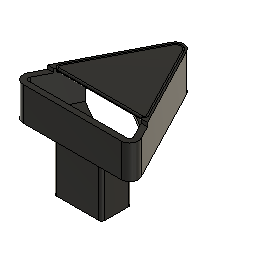
EMGmount (Autodesk Fusion 360 design; units mm, degrees)
Autodesk Fusion 360 part; units mm, degrees
sketch "Sketch5" plane through (0, 0, -6.0198) normal (0, 0, 1) x (-1, 0, 0)
  line L0 (-4.0409, -57.15) -> (2.9359, -57.15)
  line L1 (2.9359, -57.15) -> (3.9347, -56.1512)
  line L2 (3.9347, -56.1512) -> (3.9347, 6.35)
  line L3 (3.9347, 6.35) -> (-16.6393, 6.35)
  line L4 (-16.6393, 6.35) -> (-16.6393, -56.1512)
  line L5 (-16.6393, -56.1512) -> (-15.6405, -57.15)
  line L6 (-15.6405, -57.15) -> (-8.6637, -57.15)
  line L7 (-8.6637, -57.15) -> (-8.6637, -55.3466)
  arc A0 (-8.1557, -54.8386) -> (-8.6637, -55.3466) centre (-8.1557, -55.3466) ccw
  line L8 (-8.1557, -54.8386) -> (-4.5489, -54.8386)
  arc A1 (-4.0409, -55.3466) -> (-4.5489, -54.8386) centre (-4.5489, -55.3466) ccw
  line L9 (-4.0409, -55.3466) -> (-4.0409, -57.15)
  arc A2 (-8.1557, -42.1386) -> (-8.6637, -42.6466) centre (-8.1557, -42.6466) ccw
  line L10 (-8.1557, -42.1386) -> (-4.5489, -42.1386)
  arc A3 (-4.0409, -42.6466) -> (-4.5489, -42.1386) centre (-4.5489, -42.6466) ccw
  line L11 (-4.0409, -42.6466) -> (-4.0409, -46.2534)
  arc A4 (-4.5489, -46.7614) -> (-4.0409, -46.2534) centre (-4.5489, -46.2534) ccw
  line L12 (-4.5489, -46.7614) -> (-8.1557, -46.7614)
  arc A5 (-8.6637, -46.2534) -> (-8.1557, -46.7614) centre (-8.1557, -46.2534) ccw
  line L13 (-8.6637, -46.2534) -> (-8.6637, -42.6466)
  arc A6 (-8.1557, -29.4386) -> (-8.6637, -29.9466) centre (-8.1557, -29.9466) ccw
  line L14 (-8.1557, -29.4386) -> (-4.5489, -29.4386)
  arc A7 (-4.0409, -29.9466) -> (-4.5489, -29.4386) centre (-4.5489, -29.9466) ccw
  line L15 (-4.0409, -29.9466) -> (-4.0409, -33.5534)
  arc A8 (-4.5489, -34.0614) -> (-4.0409, -33.5534) centre (-4.5489, -33.5534) ccw
  line L16 (-4.5489, -34.0614) -> (-8.1557, -34.0614)
  arc A9 (-8.6637, -33.5534) -> (-8.1557, -34.0614) centre (-8.1557, -33.5534) ccw
  line L17 (-8.6637, -33.5534) -> (-8.6637, -29.9466)
  arc A10 (1.8011, -53.1114) -> (2.3091, -52.6034) centre (1.8011, -52.6034) ccw
  line L18 (1.8011, -53.1114) -> (-1.8057, -53.1114)
  arc A11 (-2.3137, -52.6034) -> (-1.8057, -53.1114) centre (-1.8057, -52.6034) ccw
  line L19 (-2.3137, -52.6034) -> (-2.3137, -48.9966)
  arc A12 (-1.8057, -48.4886) -> (-2.3137, -48.9966) centre (-1.8057, -48.9966) ccw
  line L20 (-1.8057, -48.4886) -> (1.8011, -48.4886)
  arc A13 (2.3091, -48.9966) -> (1.8011, -48.4886) centre (1.8011, -48.9966) ccw
  line L21 (2.3091, -48.9966) -> (2.3091, -52.6034)
  arc A14 (1.8011, -40.4114) -> (2.3091, -39.9034) centre (1.8011, -39.9034) ccw
  line L22 (1.8011, -40.4114) -> (-1.8057, -40.4114)
  arc A15 (-2.3137, -39.9034) -> (-1.8057, -40.4114) centre (-1.8057, -39.9034) ccw
  line L23 (-2.3137, -39.9034) -> (-2.3137, -36.2966)
  arc A16 (-1.8057, -35.7886) -> (-2.3137, -36.2966) centre (-1.8057, -36.2966) ccw
  line L24 (-1.8057, -35.7886) -> (1.8011, -35.7886)
  arc A17 (2.3091, -36.2966) -> (1.8011, -35.7886) centre (1.8011, -36.2966) ccw
  line L25 (2.3091, -36.2966) -> (2.3091, -39.9034)
  arc A18 (1.8011, -27.7114) -> (2.3091, -27.2034) centre (1.8011, -27.2034) ccw
  line L26 (1.8011, -27.7114) -> (-1.8057, -27.7114)
  arc A19 (-2.3137, -27.2034) -> (-1.8057, -27.7114) centre (-1.8057, -27.2034) ccw
  line L27 (-2.3137, -27.2034) -> (-2.3137, -23.5966)
  arc A20 (-1.8057, -23.0886) -> (-2.3137, -23.5966) centre (-1.8057, -23.5966) ccw
  line L28 (-1.8057, -23.0886) -> (1.8011, -23.0886)
  arc A21 (2.3091, -23.5966) -> (1.8011, -23.0886) centre (1.8011, -23.5966) ccw
  line L29 (2.3091, -23.5966) -> (2.3091, -27.2034)
  arc A22 (1.8011, -15.0114) -> (2.3091, -14.5034) centre (1.8011, -14.5034) ccw
  line L30 (1.8011, -15.0114) -> (-1.8057, -15.0114)
  arc A23 (-2.3137, -14.5034) -> (-1.8057, -15.0114) centre (-1.8057, -14.5034) ccw
  line L31 (-2.3137, -14.5034) -> (-2.3137, -10.8966)
  arc A24 (-1.8057, -10.3886) -> (-2.3137, -10.8966) centre (-1.8057, -10.8966) ccw
  line L32 (-1.8057, -10.3886) -> (1.8011, -10.3886)
  arc A25 (2.3091, -10.8966) -> (1.8011, -10.3886) centre (1.8011, -10.8966) ccw
  line L33 (2.3091, -10.8966) -> (2.3091, -14.5034)
  arc A26 (1.8011, -2.3114) -> (2.3091, -1.8034) centre (1.8011, -1.8034) ccw
  line L34 (1.8011, -2.3114) -> (-1.8057, -2.3114)
  arc A27 (-2.3137, -1.8034) -> (-1.8057, -2.3114) centre (-1.8057, -1.8034) ccw
  line L35 (-2.3137, -1.8034) -> (-2.3137, 1.8034)
  arc A28 (-1.8057, 2.3114) -> (-2.3137, 1.8034) centre (-1.8057, 1.8034) ccw
  line L36 (-1.8057, 2.3114) -> (1.8011, 2.3114)
  arc A29 (2.3091, 1.8034) -> (1.8011, 2.3114) centre (1.8011, 1.8034) ccw
  line L37 (2.3091, 1.8034) -> (2.3091, -1.8034)
  arc A30 (-10.8989, -53.1114) -> (-10.3909, -52.6034) centre (-10.8989, -52.6034) ccw
  line L38 (-10.8989, -53.1114) -> (-14.5057, -53.1114)
  arc A31 (-15.0137, -52.6034) -> (-14.5057, -53.1114) centre (-14.5057, -52.6034) ccw
  line L39 (-15.0137, -52.6034) -> (-15.0137, -48.9966)
  arc A32 (-14.5057, -48.4886) -> (-15.0137, -48.9966) centre (-14.5057, -48.9966) ccw
  line L40 (-14.5057, -48.4886) -> (-10.8989, -48.4886)
  arc A33 (-10.3909, -48.9966) -> (-10.8989, -48.4886) centre (-10.8989, -48.9966) ccw
  line L41 (-10.3909, -48.9966) -> (-10.3909, -52.6034)
  arc A34 (-10.8989, -40.4114) -> (-10.3909, -39.9034) centre (-10.8989, -39.9034) ccw
  line L42 (-10.8989, -40.4114) -> (-14.5057, -40.4114)
  arc A35 (-15.0137, -39.9034) -> (-14.5057, -40.4114) centre (-14.5057, -39.9034) ccw
  line L43 (-15.0137, -39.9034) -> (-15.0137, -36.2966)
  arc A36 (-14.5057, -35.7886) -> (-15.0137, -36.2966) centre (-14.5057, -36.2966) ccw
  line L44 (-14.5057, -35.7886) -> (-10.8989, -35.7886)
  arc A37 (-10.3909, -36.2966) -> (-10.8989, -35.7886) centre (-10.8989, -36.2966) ccw
  line L45 (-10.3909, -36.2966) -> (-10.3909, -39.9034)
  arc A38 (-10.8989, -27.7114) -> (-10.3909, -27.2034) centre (-10.8989, -27.2034) ccw
  line L46 (-10.8989, -27.7114) -> (-14.5057, -27.7114)
  arc A39 (-15.0137, -27.2034) -> (-14.5057, -27.7114) centre (-14.5057, -27.2034) ccw
  line L47 (-15.0137, -27.2034) -> (-15.0137, -23.5966)
  arc A40 (-14.5057, -23.0886) -> (-15.0137, -23.5966) centre (-14.5057, -23.5966) ccw
  line L48 (-14.5057, -23.0886) -> (-10.8989, -23.0886)
  arc A41 (-10.3909, -23.5966) -> (-10.8989, -23.0886) centre (-10.8989, -23.5966) ccw
  line L49 (-10.3909, -23.5966) -> (-10.3909, -27.2034)
  arc A42 (-10.8989, -15.0114) -> (-10.3909, -14.5034) centre (-10.8989, -14.5034) ccw
  line L50 (-10.8989, -15.0114) -> (-14.5057, -15.0114)
  arc A43 (-15.0137, -14.5034) -> (-14.5057, -15.0114) centre (-14.5057, -14.5034) ccw
  line L51 (-15.0137, -14.5034) -> (-15.0137, -10.8966)
  arc A44 (-14.5057, -10.3886) -> (-15.0137, -10.8966) centre (-14.5057, -10.8966) ccw
  line L52 (-14.5057, -10.3886) -> (-10.8989, -10.3886)
  arc A45 (-10.3909, -10.8966) -> (-10.8989, -10.3886) centre (-10.8989, -10.8966) ccw
  line L53 (-10.3909, -10.8966) -> (-10.3909, -14.5034)
  arc A46 (-10.8989, -2.3114) -> (-10.3909, -1.8034) centre (-10.8989, -1.8034) ccw
  line L54 (-10.8989, -2.3114) -> (-14.5057, -2.3114)
  arc A47 (-15.0137, -1.8034) -> (-14.5057, -2.3114) centre (-14.5057, -1.8034) ccw
  line L55 (-15.0137, -1.8034) -> (-15.0137, 1.8034)
  arc A48 (-14.5057, 2.3114) -> (-15.0137, 1.8034) centre (-14.5057, 1.8034) ccw
  line L56 (-14.5057, 2.3114) -> (-10.8989, 2.3114)
  arc A49 (-10.3909, 1.8034) -> (-10.8989, 2.3114) centre (-10.8989, 1.8034) ccw
  line L57 (-10.3909, 1.8034) -> (-10.3909, -1.8034)
  arc A50 (-8.6637, -8.1534) -> (-8.1557, -8.6614) centre (-8.1557, -8.1534) ccw
  line L58 (-8.6637, -8.1534) -> (-8.6637, -4.5466)
  arc A51 (-8.1557, -4.0386) -> (-8.6637, -4.5466) centre (-8.1557, -4.5466) ccw
  line L59 (-8.1557, -4.0386) -> (-4.5489, -4.0386)
  arc A52 (-4.0409, -4.5466) -> (-4.5489, -4.0386) centre (-4.5489, -4.5466) ccw
  line L60 (-4.0409, -4.5466) -> (-4.0409, -8.1534)
  arc A53 (-4.5489, -8.6614) -> (-4.0409, -8.1534) centre (-4.5489, -8.1534) ccw
  line L61 (-4.5489, -8.6614) -> (-8.1557, -8.6614)
  arc A54 (-8.1557, -16.7386) -> (-8.6637, -17.2466) centre (-8.1557, -17.2466) ccw
  line L62 (-8.1557, -16.7386) -> (-4.5489, -16.7386)
  arc A55 (-4.0409, -17.2466) -> (-4.5489, -16.7386) centre (-4.5489, -17.2466) ccw
  line L63 (-4.0409, -17.2466) -> (-4.0409, -20.8534)
  arc A56 (-4.5489, -21.3614) -> (-4.0409, -20.8534) centre (-4.5489, -20.8534) ccw
  line L64 (-4.5489, -21.3614) -> (-8.1557, -21.3614)
  arc A57 (-8.6637, -20.8534) -> (-8.1557, -21.3614) centre (-8.1557, -20.8534) ccw
  line L65 (-8.6637, -20.8534) -> (-8.6637, -17.2466)
  line L66 (3.9347, 5.08) -> (3.9347, -5.08)
  line L67 (2.6647, -6.35) -> (-15.3693, -6.35)
  line L68 (-16.6393, -5.08) -> (-16.6393, 5.08)
  line L69 (-15.3693, 6.35) -> (2.6647, 6.35)
  arc A58 (2.6647, -6.35) -> (3.9347, -5.08) centre (2.6647, -5.08) ccw
  arc A59 (3.9347, 5.08) -> (2.6647, 6.35) centre (2.6647, 5.08) ccw
  arc A60 (-16.6393, -5.08) -> (-15.3693, -6.35) centre (-15.3693, -5.08) ccw
  arc A61 (-15.3693, 6.35) -> (-16.6393, 5.08) centre (-15.3693, 5.08) ccw
  point P0 (3.9347, 6.35)
  point P1 (3.9347, -6.35)
  dimension "d56" = 12.7
  dimension "d57" = 1.27
  constraint coincident P0 L2.end
  constraint coincident L2 P1
  constraint perpendicular L4 L67
  constraint coincident P1 L66
  constraint coincident P1 L67
  constraint tangent L66 A58
  constraint tangent L67 A58
  constraint coincident P0 L66
  constraint coincident P0 L69
  constraint tangent L66 A59
  constraint tangent L69 A59
  constraint equal A58 A59
  constraint tangent L67 A60
  constraint tangent L68 A60
  constraint equal A58 A60
  constraint tangent L68 A61
  constraint tangent L69 A61
  constraint equal A58 A61
  measures "d56" distance of P0 P1
  measures "d57" radius of A58
extrude "Extrude8" add sketch "Sketch5" along normal blind 22.225 contours L2 L3 L4 L58 A51 L59 A52 L60 L66 L67 L68 L69 A58 A59 A60 A61 | L58 A51 L59 A52 L60 L67 | A26 L34 A27 L35 A28 L36 A29 L37 | A46 L54 A47 L55 A48 L56 A49 L57 makes body 1
sketch "Sketch9" plane through (0, 0, 16.2052) normal (0, 0, 1) x (-1, 0, 0)
  arc A0 (3.9347, 5.08) -> (2.6647, 6.35) centre (2.6647, 5.08) ccw
  line L0 (2.6647, 6.35) -> (-15.3693, 6.35)
  arc A1 (-15.3693, 6.35) -> (-16.6393, 5.08) centre (-15.3693, 5.08) ccw
  line L1 (-16.6393, 5.08) -> (-16.6393, -5.08)
  arc A2 (-16.6393, -5.08) -> (-15.3693, -6.35) centre (-15.3693, -5.08) ccw
  line L2 (-15.3693, -6.35) -> (2.6647, -6.35)
  arc A3 (2.6647, -6.35) -> (3.9347, -5.08) centre (2.6647, -5.08) ccw
  line L3 (3.9347, -5.08) -> (3.9347, 5.08)
  line L4 (-6.3523, 6.35) -> (-27.2641, 6.35)
  line L5 (-6.3523, 6.35) -> (14.5594, 6.35)
  line L6 (-6.3523, 6.35) -> (-6.3523, -83.9563)
  line L7 (15.6871, 4.4958) -> (-5.2247, -35.8693)
  line L8 (-7.48, -35.8693) -> (-28.3917, 4.4958)
  arc A4 (-7.48, -35.8693) -> (-5.2247, -35.8693) centre (-6.3523, -35.2851) ccw
  arc A5 (-27.2641, 6.35) -> (-28.3917, 4.4958) centre (-27.2641, 5.08) ccw
  arc A6 (15.6871, 4.4958) -> (14.5594, 6.35) centre (14.5594, 5.08) ccw
  line L9 (-6.3523, 8.7312) -> (-27.2641, 8.7312)
  arc A7 (-27.2641, 8.7312) -> (-30.5061, 3.4004) centre (-27.2641, 5.08) ccw
  line L10 (-9.5943, -36.9647) -> (-30.5061, 3.4004)
  arc A8 (-9.5943, -36.9647) -> (-3.1103, -36.9647) centre (-6.3523, -35.2851) ccw
  line L11 (17.8014, 3.4004) -> (-3.1103, -36.9647)
  arc A9 (17.8014, 3.4004) -> (14.5594, 8.7313) centre (14.5594, 5.08) ccw
  line L12 (-6.3523, 8.7312) -> (14.5594, 8.7312)
  point P0 (-29.3523, 6.35)
  point P1 (16.6477, 6.35)
  point P2 (-6.3523, -38.0459)
  dimension "d100" = 23
  dimension "d101" = 23
  dimension "d102" = 50
  dimension "d103" = 1.27
  dimension "d104" = -2.3813
  constraint midpoint L0 L4.start
  constraint parallel L0 L4
  constraint parallel L0 L5
  constraint perpendicular L5 L6
  constraint coincident L6 P2
  constraint coincident P2 L7
  constraint coincident P2 L8
  constraint tangent L7 A4
  constraint tangent L8 A4
  constraint coincident P0 L4
  constraint coincident P0 L8
  constraint tangent L4 A5
  constraint tangent L8 A5
  constraint equal A4 A5
  constraint coincident P1 L5
  constraint coincident P1 L7
  constraint tangent L5 A6
  constraint tangent L7 A6
  constraint equal A4 A6
  measures "d100" distance of L4.start P0
  measures "d101" distance of L4.start P1
  measures "d102" distance of P1 P2
  measures "d103" radius of A4
extrude "Extrude15" add sketch "Sketch9" along normal blind 14.2875 separate body makes body 2
extrude "Extrude16" add sketch "Sketch9" along normal blind 1.5875 contours A0 L0 L2 A3 L3 L5 L6 | A0 L2 A3 L3 L5 L6 L7 A4 A6 | L0 A1 L1 A2 L2 L4 L6 | A1 L1 A2 L2 L4 L6 L8 A4 A5 bodies 1 2
sketch "Sketch10" plane through (0, 0, 16.2052) normal (0, 0, -1) x (1, 0, 0)
  arc A0 (16.6393, 5.08) -> (15.3693, 6.35) centre (15.3693, 5.08) ccw
  line L0 (16.6393, 5.08) -> (16.6393, -5.08)
  arc A1 (15.3693, -6.35) -> (16.6393, -5.08) centre (15.3693, -5.08) ccw
  line L1 (15.3693, -6.35) -> (-2.6647, -6.35)
  arc A2 (-3.9347, -5.08) -> (-2.6647, -6.35) centre (-2.6647, -5.08) ccw
  line L2 (-3.9347, -5.08) -> (-3.9347, 5.08)
  arc A3 (-2.6647, 6.35) -> (-3.9347, 5.08) centre (-2.6647, 5.08) ccw
  line L3 (-2.6647, 6.35) -> (15.3693, 6.35)
  arc A4 (30.5061, 3.4004) -> (27.2641, 8.7312) centre (27.2641, 5.08) ccw
  line L4 (27.2641, 8.7312) -> (-14.5594, 8.7312)
  arc A5 (-14.5594, 8.7312) -> (-17.8014, 3.4004) centre (-14.5594, 5.08) ccw
  line L5 (-17.8014, 3.4004) -> (3.1103, -36.9647)
  arc A6 (3.1103, -36.9647) -> (9.5943, -36.9647) centre (6.3523, -35.2851) ccw
  line L6 (9.5943, -36.9647) -> (30.5061, 3.4004)
  line L7 (7.0603, -44.5891) -> (-20.7698, 9.13)
  line L8 (-6.8547, -17.7295) -> (15.1423, -5.0295)
  line L9 (-6.8547, -17.7295) -> (11.4408, -17.7295) construction
  line L10 (15.1423, -5.0295) -> (12.6023, -0.6301)
  line L11 (10.8674, -0.1653) -> (-9.7788, -12.0854)
  line L12 (15.1423, -5.0295) -> (17.6823, -9.4289)
  line L13 (17.2174, -11.1638) -> (-3.9307, -23.3737)
  line L14 (-3.9307, -23.3737) -> (-9.7788, -12.0854)
  arc A7 (17.2174, -11.1638) -> (17.6823, -9.4289) centre (16.5824, -10.0639) ccw
  arc A8 (12.6023, -0.6301) -> (10.8674, -0.1653) centre (11.5024, -1.2651) ccw
  point P0 (11.9673, 0.4697)
  point P1 (18.3173, -10.5288)
  dimension "d109" = 30
  dimension "d110" = 25.4
  dimension "d111" = 6.35
  dimension "d112" = 90
  dimension "d113" = 6.35
  dimension "d114" = 90
  dimension "d115" = 1.27
  constraint parallel L5 L7
  constraint horizontal L9
  constraint midpoint L7 L8.start
  constraint perpendicular L8 L10
  constraint coincident L5 L11.end
  constraint coincident L7 L11.end
  constraint perpendicular L8 L12
  constraint coincident L7 L13.end
  constraint coincident P1 L12
  constraint coincident P1 L13
  constraint tangent L12 A7
  constraint tangent L13 A7
  constraint coincident P0 L10
  constraint coincident P0 L11
  constraint tangent L10 A8
  constraint tangent L11 A8
  constraint equal A7 A8
  measures "d109" angle of L8 L9
  measures "d110" distance of L8.start L8.end
  measures "d111" distance of L8.end P0
  measures "d112" angle of L10 L11
  measures "d113" distance of L8.end P1
  measures "d114" angle of L12 L13
  measures "d115" radius of A7
extrude "Extrude17" cut sketch "Sketch10" against normal blind 1.6002 contours A1 L1 L5 L7 L8 L12 L13 L14 A7 | A1 L1 L8 L12 | L1 L8 L10 L11 A8 | L1 L5 L7 L8 L11 L14 bodies 1
extrude "Extrude18" cut sketch "Sketch10" along normal blind 9.525 contours A1 L1 L5 L7 L8 L12 L13 L14 A7 | A1 L1 L8 L12 | L1 L8 L10 L11 A8 | L1 L5 L7 L8 L11 L14 bodies 1
sketch "Sketch11" plane through (0, 0, 30.4927) normal (0, 0, 1) x (-1, 0, 0)
  arc A0 (-7.48, -35.8693) -> (-5.2247, -35.8693) centre (-6.3523, -35.2851) ccw
  line L0 (-7.48, -35.8693) -> (-28.3917, 4.4958)
  arc A1 (-27.2641, 6.35) -> (-28.3917, 4.4958) centre (-27.2641, 5.08) ccw
  line L1 (-27.2641, 6.35) -> (14.5594, 6.35)
  arc A2 (15.6871, 4.4958) -> (14.5594, 6.35) centre (14.5594, 5.08) ccw
  line L2 (15.6871, 4.4958) -> (-5.2247, -35.8693)
  arc A3 (-27.2641, 8.7312) -> (-30.5061, 3.4004) centre (-27.2641, 5.08) ccw
  line L3 (-30.5061, 3.4004) -> (-9.5943, -36.9647)
  arc A4 (-9.5943, -36.9647) -> (-3.1103, -36.9647) centre (-6.3523, -35.2851) ccw
  line L4 (-3.1103, -36.9647) -> (17.8014, 3.4004)
  arc A5 (17.8014, 3.4004) -> (14.5594, 8.7313) centre (14.5594, 5.08) ccw
  line L5 (14.5594, 8.7313) -> (-27.2641, 8.7312)
  line L6 (20.7799, 9.1479) -> (14.9379, -2.1287)
  line L7 (14.9379, -2.1287) -> (-27.6416, -2.1287)
  line L8 (14.9379, -2.1287) -> (-3.1099, -36.9655)
  line L9 (-9.5939, -36.9655) -> (-27.6416, -2.1287)
  arc A6 (-9.5939, -36.9655) -> (-3.1099, -36.9655) centre (-6.3519, -35.2859) ccw
  line L10 (12.6721, -4.7766) -> (-3.8147, -36.6004)
  arc A7 (-8.8891, -36.6004) -> (-3.8147, -36.6004) centre (-6.3519, -35.2859) ccw
  line L11 (-8.8891, -36.6004) -> (-25.3759, -4.7766)
  line L12 (11.5445, -2.9224) -> (-24.2482, -2.9224)
  arc A8 (12.6721, -4.7766) -> (11.5445, -2.9224) centre (11.5445, -4.1924) ccw
  arc A9 (-24.2482, -2.9224) -> (-25.3759, -4.7766) centre (-24.2482, -4.1924) ccw
  line L13 (11.8274, -2.9544) -> (12.2552, -2.1287)
  line L14 (-24.532, -2.9545) -> (-24.9598, -2.1287)
  dimension "d122" = 12.7
  dimension "d123" = 3.6513
  dimension "d125" = 1.27
  constraint parallel L4 L6
  constraint coincident L3 L7.end
  constraint horizontal L7
  constraint parallel L4 L8
  constraint parallel L3 L9
  constraint tangent L8 A6
  constraint tangent L9 A6
  constraint concentric A6 A7
  constraint tangent L10 A7
  constraint tangent A7 L11
  constraint tangent L10 A8
  constraint tangent L12 A8
  constraint tangent L11 A9
  constraint tangent L12 A9
  constraint equal A8 A9
  constraint coincident A8 L13.start
  constraint coincident L2 L13.start
  constraint coincident L7 L13.end
  constraint coincident L2 L13.end
  constraint coincident A9 L14.start
  constraint coincident L0 L14.start
  constraint coincident L7 L14.end
  constraint coincident L0 L14.end
  measures "d122" distance of L6.start L6.end
  measures "d123" radius of A6
  measures "d125" radius of A8
extrude "Extrude19" add sketch "Sketch11" along normal blind 1.5875 contours L0 L2 L3 A4 L4 L7 L8 L9 A6 L10 A7 L11 A8 A9 L13 L14 bodies 1
extrude "Extrude20" add sketch "Sketch11" along normal blind 1.5875 separate body contours A0 L0 L2 L12 A8 A9 | A0 L0 L2 L10 A7 L11 A8 A9 makes body 3
move_body "Move5" bodies 3 to x (1, 0, 0) y (0, 1, 0) z (0, 0, 1) at (0, 0, 12.7)
fillet "Fillet8" radius 0.635 12 edges at (17.1325, 20.6885, 44.7802) (6.3519, 38.1434, 44.7802) (-4.4287, 20.6885, 44.7802) (-12.6295, 3.5325, 44.7802) (6.3519, 2.9224, 44.7802) (25.3333, 3.5325, 44.7802) (17.1325, 20.6885, 43.1927) (6.3519, 38.1434, 43.1927) (-4.4287, 20.6885, 43.1927) (-12.6295, 3.5325, 43.1927) (6.3519, 2.9224, 43.1927) (25.3333, 3.5325, 43.1927) on bodies 3
move_body "Move6" bodies 3 to x (1, 0, 0) y (0, 1, 0) z (0, 0, 1) at (0, 0, -12.7)
hole "Hole5" at (12.7, 0, -6.0198) direction (0, 0, 1) diameter 3.429 depth 10.16 tip angle 180 bodies 1
thread "Thread5" "ANSI Unified Screw Threads 0.164(#8) 8-32 UNC 8-32 UNC 2B" major diameter 4.1656 minor diameter 3.4163 pitch 0.7937 angle 60 modelled right hand crest width 0.2341 on face at (12.7855, 1.7124, -2.6331) crest through (10.9919, 0, -5.8214) on bodies 1
hole "Hole6" at (0, 0, -6.0198) direction (0, 0, 1) diameter 3.429 depth 10.16 tip angle 180 bodies 1
thread "Thread6" "ANSI Unified Screw Threads 0.164(#8) 8-32 UNC 8-32 UNC 2B" major diameter 4.1656 minor diameter 3.4163 pitch 0.7937 angle 60 modelled right hand crest width 0.2341 on face at (0.0855, 1.7124, -2.6331) crest through (-1.7081, 0, -5.8214) on bodies 1
extrude "Extrude21" cut sketch "Sketch10" against normal blind 6.35 contours A1 L1 L5 L7 L8 L12 L13 L14 A7 | A1 L1 L8 L12 | L1 L8 L10 L11 A8 | L1 L5 L7 L8 L11 L14 bodies 1
equation "d58 = ( 7 / 8 ) * 1 in"
equation "d104 = ( -3 / 32 ) * 1 in"
equation "d105 = ( 1 / 16 ) * 1 in + ( 1 / 2 ) * 1 in"
equation "d107 = ( 1 / 16 ) * 1 in"
equation "d118 = ( 3 / 8 ) * 1 in"
equation "d126 = ( 1 / 16 ) * 1 in"
equation "d128 = ( 1 / 16 ) * 1 in"
equation "d142 = ( -1 / 4 ) * 1 in"
named bodies: "EMGmount", "EMGcover"
